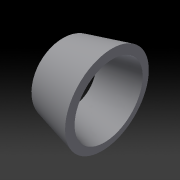
# Autodesk Inventor part: Beveled Sleeve
Saved by Autodesk Inventor 2016 (Build 200138000, 138)
## iProperties
Created: 2012-08-08
Part Number: Beveled Sleeve
Material: Generic
Document SubType Name: Modeling
Designer: John
Density: 1 g/cm^3
Appearance: Default
Author: John
Autodesk Inventor part; units mm, degrees
ref_plane "XZ Plane" through (0, 0, 0) normal (0, 1, 0) x (-1, 0, 0)
ref_plane "XY Plane" through (0, 0, 0) normal (0, 0, 1) x (1, 0, 0)
sketch "Sketch1" plane through (0, 0, 0) normal (1, 0, 0) x (0, 1, 0)
  circle A0 centre (0, 0) radius 4.826
  dimension "d0" = 9.652
  constraints: 1 centre point, 1 coincident
  measures "d0" diameter of A0
ref_plane "Work Plane1" through (-4.8514, 0, 0) normal (1, 0, 0) x (0, 1, 0)
sketch "Sketch2" plane through (-4.8514, 0, 0) normal (1, 0, 0) x (0, 1, 0)
  circle A0 centre (0, 0) radius 4.1275
  dimension "d2" = 8.255
  constraints: 1 centre point, 1 coincident
  measures "d2" diameter of A0
loft "Loft1" add profiles "Sketch1", "Sketch2"
shell "Shell1" thickness 0.8636 removed faces 2 at (0, 1.0666, -0.7041) at (-4.8514, -0.4879, 1.9449)
body "Solid1"
